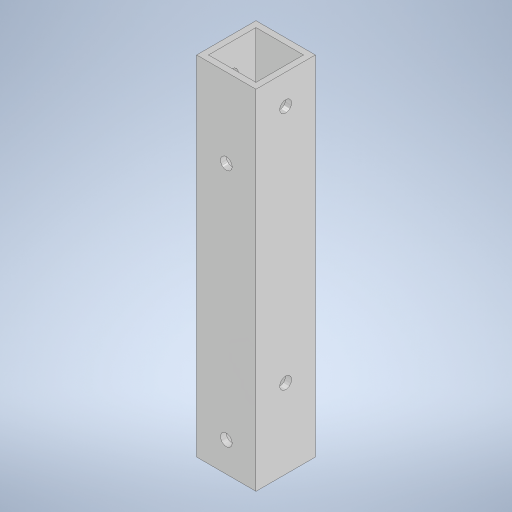
# Autodesk Inventor part: omu_k_jo_11
Saved by Autodesk Inventor 2024.2 (Build 282272000, 272)
## iProperties
Created: 2024-01-23
Part Number: omu_k_jo_11
Material: アルミニウム 6061-AHC
Document SubType Name: Modeling
Designer: fhbdh
Density: 2.7 g/cm^3
Appearance: アルミニウム - ダーク
Author: fhbdh
Autodesk Inventor part; units mm, degrees
ref_plane "YZ Plane" through (0, 0, 0) normal (1, 0, 0) x (0, 1, 0)
ref_plane "XZ Plane" through (0, 0, 0) normal (0, 1, 0) x (-1, 0, 0)
ref_plane "XY Plane" through (0, 0, 0) normal (0, 0, 1) x (1, 0, 0)
sketch "スケッチ1" plane through (0, 0, 0) normal (0, 1, 0) x (-1, 0, 0)
  line L0 (7.5, -7.5) -> (-7.5, -7.5)
  line L1 (-7.5, -7.5) -> (-7.5, 7.5)
  line L2 (-7.5, 7.5) -> (7.5, 7.5)
  line L3 (7.5, 7.5) -> (7.5, -7.5)
  line L4 (7.5, -7.5) -> (-7.5, 7.5) construction
  line L5 (-7.5, -7.5) -> (7.5, 7.5) construction
  line L6 (6, -6) -> (-6, -6)
  line L7 (-6, -6) -> (-6, 6)
  line L8 (-6, 6) -> (6, 6)
  line L9 (6, 6) -> (6, -6)
  point P0 (0, 0)
  dimension "d0" = 15
  dimension "d1" = 15
  dimension "d2" = 1.5
  constraints: 20 end point, 4 parallel, 2 midpoint, 2 perpendicular, 1 horizontal, 3 other
  measures "d0" distance of L1.end L2.end
  measures "d1" distance of L2.end L0.start
  measures "d2" distance between parallel lines of L3 L9
extrude "押し出し1" add sketch "スケッチ1" along normal blind 88
sketch "スケッチ2" plane through (-7.5, 0, 7.5) normal (0, 0, 1) x (1, 0, 0)
  line L0 (7.5, 0) -> (7.5, 88) construction
  line L1 (0, 88) -> (15, 88) projected
  line L2 (0, 0) -> (0, 88) projected
  line L3 (0, 44) -> (15, 44) construction
  line L4 (15, 0) -> (15, 88) projected
  constraints: 4 end point, 3 midpoint
sketch "スケッチ3" plane through (7.5, 0, 7.5) normal (1, 0, 0) x (0, 0, -1)
  line L0 (7.5, 0) -> (7.5, 88) construction
  line L1 (0, 88) -> (15, 88) projected
  line L2 (15, 0) -> (15, 88) projected
  line L3 (15, 44) -> (0, 44) construction
  line L4 (0, 0) -> (0, 88) projected
  constraints: 4 end point, 3 midpoint
sketch "スケッチ4" plane through (-7.5, 0, 7.5) normal (0, 0, 1) x (1, 0, 0)
  line L0 (7.5, 0) -> (7.5, 88) construction
  circle A0 centre (7.5, 7.5) radius 1.5
  line L1 (0, 0) -> (15, 0) projected
  circle A1 centre (7.5, 68) radius 1.5
  line L2 (0, 88) -> (15, 88) projected
  dimension "d5" = 3
  dimension "d6" = 7.5
  dimension "d13" = 3
  dimension "d14" = 20
  constraints: 2 centre point, 2 point on line
  measures "d5" diameter of A0
  measures "d6" distance from line of L1 A0.centre
  measures "d13" diameter of A1
  measures "d14" distance from line of L2 A1.centre
extrude "押し出し2" cut sketch "スケッチ4" against normal through all
sketch "スケッチ5" plane through (7.5, 0, 7.5) normal (1, 0, 0) x (0, 0, -1)
  circle A0 centre (7.5, 20) radius 1.5
  line L0 (7.5, 0) -> (7.5, 88) construction
  line L1 (0, 0) -> (15, 0) projected
  circle A1 centre (7.5, 80.5) radius 1.5
  line L2 (0, 88) -> (15, 88) projected
  dimension "d9" = 3
  dimension "d10" = 20
  dimension "d15" = 3
  dimension "d16" = 7.5
  constraints: 2 centre point, 2 point on line
  measures "d9" diameter of A0
  measures "d10" distance from line of L1 A0.centre
  measures "d15" diameter of A1
  measures "d16" distance from line of L2 A1.centre
extrude "押し出し3" cut sketch "スケッチ5" against normal through all
sketch "スケッチ6" plane through (7.5, 0, 7.5) normal (1, 0, 0) x (0, 0, -1)
  circle A0 centre (7.5, 80.5) radius 1.5 projected
  line L0 (0, 88) -> (15, 88) projected
  circle A1 centre (7.5, 20) radius 1.5 projected
  line L1 (0, 0) -> (15, 0) projected
  point P0 (7.5, 0)
  dimension "d17" = 7.5
  dimension "d18" = 68
  dimension "d19" = 88
  measures "d17" distance from line of A0.centre L0
  measures "d18" distance from line of A1.centre L0
  measures "d19" distance between parallel lines of L1 L0
sketch "スケッチ7" plane through (-7.5, 0, 7.5) normal (0, 0, 1) x (1, 0, 0)
  circle A0 centre (7.5, 68) radius 1.5 projected
  line L0 (0, 88) -> (15, 88) projected
  circle A1 centre (7.5, 7.5) radius 1.5 projected
  point P0 (7.5, 0)
  dimension "d20" = 20
  dimension "d21" = 80.5
  measures "d20" distance from line of A0.centre L0
  measures "d21" distance from line of A1.centre L0
equation "\"d1\" = d0"
